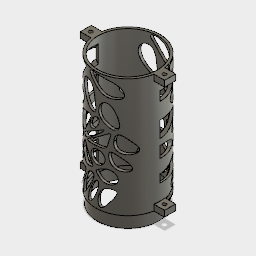
MIDDLEv2 v0XXX (Autodesk Fusion 360 design; units mm, degrees)
Autodesk Fusion 360 part; units mm, degrees
note: some values were not read from the file. Chosen so that the rebuilt part matches the saved one: that a step has no effect; which bodies a step acts on.
(part 1 of 3)
sketch "Sketch1" plane through (0, 0, 0) normal (0, 1, 0) x (1, 0, 0)
  circle A0 centre (0, 0) radius 25
  circle A1 centre (0, 0) radius 27
  circle A2 centre (0, 0) radius 26
  line L0 (-26.5898, 4.6885) -> (-35.5898, 4.6885)
  line L1 (-26.5898, -4.6885) -> (-35.5898, -4.6885)
  line L2 (-35.5898, 4.6885) -> (-35.5898, -4.6885)
  line L3 (0, 0) -> (26.3565, 0) construction
  line L4 (26.5898, 4.6885) -> (35.5898, 4.6885)
  line L5 (26.5898, -4.6885) -> (35.5898, -4.6885)
  line L6 (35.5898, -4.6885) -> (35.5898, 4.6885)
  line L7 (35.5898, 4.6885) -> (35.5898, -0.3115)
  line L8 (35.5898, -0.3115) -> (31.0898, -0.3115)
  line L9 (-35.5898, 4.6885) -> (-35.5898, -0.3115)
  line L10 (-35.5898, -0.3115) -> (-31.0898, -0.3115)
  circle A3 centre (-31.0898, -0.3115) radius 1.5
  circle A4 centre (31.0898, -0.3115) radius 1.5
extrude "Extrude1" add sketch "Sketch1" against normal blind 10 contours A2 makes body 1
extrude "Extrude2" add sketch "Sketch1" along normal blind 100 separate body contours A1 | A2 makes body 2
extrude "Extrude3" add sketch "Sketch1" along normal blind 5 separate body contours A1 L4 L5 L6 L7 | A1 L0 L1 L2 L9 makes body 3 at (31.0524, 5, -3.5204) makes body 4 at (-31.1272, 0, -3.5204)
extrude "Extrude4" cut 1 faces at (31.0524, 5, -3.5204) along direction (0, -1, 0) blind 5 on bodies 3 bodies 3
extrude "Extrude5" add sketch "Sketch1" along normal blind 100 contours A1 L4 L5 L6 L7 bodies 1 2 4
extrude "Extrude6" cut sketch "Sketch1" along normal blind 95 contours A1 L4 L5 L6 L7 bodies 2
extrude "Extrude7" add sketch "Sketch1" along normal blind 5 contours A1 L4 L5 L6 L7 bodies 2
extrude "Extrude8" cut sketch "Sketch1" along normal blind 5 contours A1 L0 L1 L2 L9 bodies 4
extrude "Extrude9" add sketch "Sketch1" along normal blind 100 contours A1 L0 L1 L2 L9 bodies 1 2
extrude "Extrude10" cut sketch "Sketch1" along normal blind 95 contours A1 L0 L1 L2 L9 bodies 2
extrude "Extrude11" add sketch "Sketch1" along normal blind 5 contours A1 L0 L1 L2 L9 bodies 2
replace_face "ReplaceFace1" [no effect]
mesh "Mesh1" [no effect]
sketch "Voronoi - Sketch2" plane through (0, 0, 0) normal (0, 0, 1) x (1, 0, 0)
  spline S0 degree 5 poles (72.3415, 4.2484) (72.4082, 4.3865) (72.5984, 4.6454) (73.0509, 4.9752) (73.962, 5.2758) (75.4951, 5.3871) (77.2684, 5.2236) (79.1091, 4.7979) (80.8407, 4.1464) (82.2997, 3.3318) (83.3471, 2.4369) (83.8777, 1.5524) (83.8316, 0.7678) (83.2057, 0.1602) (82.0668, -0.2155) (80.5337, -0.3268) (78.7604, -0.1633) (76.9197, 0.2623) (75.1881, 0.9139) (73.7291, 1.7284) (72.6817, 2.6234) (72.2572, 3.3309) (72.1984, 3.8167) (72.2749, 4.1103) (72.3415, 4.2484) knots 0 0 0 0 0 0 0.05 0.1 0.15 0.2 0.25 0.3 0.35 0.4 0.45 0.5 0.55 0.6 0.65 0.7 0.75 0.8 0.85 0.9 0.95 1 1 1 1 1 1
  spline S1 degree 5 poles (46.3148, 2.7293) (46.337, 2.8682) (46.4367, 3.1463) (46.7508, 3.5578) (47.4808, 4.0684) (48.815, 4.5828) (50.4367, 4.9223) (52.1886, 5.0509) (53.9042, 4.9524) (55.421, 4.6371) (56.5931, 4.1395) (57.3025, 3.5104) (57.4721, 2.8117) (57.0782, 2.1102) (56.1658, 1.4718) (54.8316, 0.9575) (53.2099, 0.618) (51.4579, 0.4893) (49.7424, 0.5878) (48.2256, 0.9031) (47.0535, 1.4008) (46.4859, 1.904) (46.3032, 2.3128) (46.2925, 2.5904) (46.3148, 2.7293) knots 0 0 0 0 0 0 0.05 0.1 0.15 0.2 0.25 0.3 0.35 0.4 0.45 0.5 0.55 0.6 0.65 0.7 0.75 0.8 0.85 0.9 0.95 1 1 1 1 1 1
  spline S2 degree 5 poles (90.4982, 7.9713) (90.7384, 8.2375) (91.2179, 8.7662) (91.9267, 9.5441) (92.8297, 10.5357) (93.8765, 11.6727) (94.8535, 12.6841) (95.7813, 13.5418) (96.6728, 14.207) (97.5157, 14.6194) (98.2635, 14.6976) (98.8599, 14.3734) (99.2596, 13.6216) (99.4483, 12.4904) (99.432, 11.0769) (99.2268, 9.5051) (98.8489, 7.9027) (98.3044, 6.3793) (97.579, 5.0034) (96.6518, 3.8123) (95.5082, 2.8218) (94.1538, 2.035) (92.6267, 1.4513) (91.0135, 1.0766) (89.4568, 0.9294) (88.1201, 1.0316) (87.1574, 1.4004) (86.6833, 2.0404) (86.7368, 2.9339) (87.2654, 4.0371) (88.1609, 5.2904) (89.0607, 6.3596) (89.7768, 7.1693) (90.258, 7.7052) (90.4982, 7.9713) knots 0 0 0 0 0 0 0.033333 0.066667 0.1 0.133333 0.166667 0.2 0.233333 0.266667 0.3 0.333333 0.366667 0.4 0.433333 0.466667 0.5 0.533333 0.566667 0.6 0.633333 0.666667 0.7 0.733333 0.766667 0.8 0.833333 0.866667 0.9 0.933333 0.966667 1 1 1 1 1 1
  spline S3 degree 5 poles (41.8576, 8.6332) (42.0475, 9.0262) (42.4323, 9.8124) (43.0168, 10.976) (43.7881, 12.4263) (44.7081, 13.9003) (45.5694, 14.8884) (46.3642, 15.2901) (47.083, 15.0691) (47.7037, 14.2835) (48.1907, 13.0747) (48.5028, 11.6193) (48.598, 10.0934) (48.4404, 8.6303) (48.0059, 7.285) (47.2874, 6.0631) (46.3009, 4.9442) (45.0912, 3.9084) (43.7371, 2.9591) (42.3613, 2.153) (41.1092, 1.5828) (40.1213, 1.3501) (39.5091, 1.5424) (39.3259, 2.2057) (39.55, 3.3263) (40.1114, 4.8434) (40.7519, 6.2937) (41.2925, 7.4546) (41.6676, 8.2403) (41.8576, 8.6332) knots 0 0 0 0 0 0 0.04 0.08 0.12 0.16 0.2 0.24 0.28 0.32 0.36 0.4 0.44 0.48 0.52 0.56 0.6 0.64 0.68 0.72 0.76 0.8 0.84 0.88 0.92 0.96 1 1 1 1 1 1
  spline S4 degree 5 poles (51.1992, 14.78) (51.3166, 14.7901) (51.5593, 14.7689) (51.9419, 14.6132) (52.4643, 14.1659) (53.0742, 13.268) (53.58, 12.1218) (53.93, 10.8378) (54.0877, 9.5375) (54.0399, 8.3441) (53.7944, 7.3733) (53.3764, 6.7228) (52.8255, 6.4623) (52.1932, 6.6219) (51.5401, 7.1811) (50.9302, 8.079) (50.4244, 9.2252) (50.0744, 10.5091) (49.9167, 11.8095) (49.9645, 13.0028) (50.21, 13.9737) (50.5444, 14.494) (50.855, 14.7088) (51.0818, 14.77) (51.1992, 14.78) knots 0 0 0 0 0 0 0.05 0.1 0.15 0.2 0.25 0.3 0.35 0.4 0.45 0.5 0.55 0.6 0.65 0.7 0.75 0.8 0.85 0.9 0.95 1 1 1 1 1 1
  spline S5 degree 5 poles (76.6274, 11.9383) (76.6372, 12.173) (76.695, 12.6311) (76.8959, 13.2798) (77.3869, 14.0619) (78.3402, 14.9156) (79.5819, 15.6646) (81.0431, 16.3133) (82.6365, 16.8224) (84.2611, 17.1145) (85.8113, 17.1022) (87.1843, 16.7107) (88.2878, 15.9002) (89.0488, 14.6948) (89.4192, 13.1895) (89.3745, 11.5212) (88.9153, 9.8484) (88.0682, 8.3286) (86.8872, 7.0949) (85.4537, 6.2384) (83.866, 5.8125) (82.2311, 5.8331) (80.6564, 6.2796) (79.2407, 7.0949) (78.0656, 8.1849) (77.195, 9.4353) (76.7786, 10.4711) (76.6361, 11.2226) (76.6176, 11.7035) (76.6274, 11.9383) knots 0 0 0 0 0 0 0.04 0.08 0.12 0.16 0.2 0.24 0.28 0.32 0.36 0.4 0.44 0.48 0.52 0.56 0.6 0.64 0.68 0.72 0.76 0.8 0.84 0.88 0.92 0.96 1 1 1 1 1 1
  spline S6 degree 5 poles (63.4479, 5.5707) (63.4765, 5.8196) (63.5586, 6.3186) (63.7559, 7.0631) (64.1633, 8.0259) (64.8897, 9.157) (65.799, 10.2126) (66.848, 11.1957) (67.9864, 12.1029) (69.1584, 12.9105) (70.3047, 13.5634) (71.367, 13.9945) (72.2924, 14.1422) (73.0371, 13.9685) (73.5718, 13.4785) (73.8847, 12.7343) (73.9769, 11.8229) (73.858, 10.8318) (73.5415, 9.8153) (73.0424, 8.7851) (72.3787, 7.7324) (71.5719, 6.6433) (70.6476, 5.5163) (69.6371, 4.3784) (68.5773, 3.305) (67.5102, 2.3997) (66.48, 1.772) (65.5316, 1.514) (64.7086, 1.6806) (64.0514, 2.2613) (63.5952, 3.1783) (63.4129, 4.0923) (63.3868, 4.8254) (63.4193, 5.3218) (63.4479, 5.5707) knots 0 0 0 0 0 0 0.033333 0.066667 0.1 0.133333 0.166667 0.2 0.233333 0.266667 0.3 0.333333 0.366667 0.4 0.433333 0.466667 0.5 0.533333 0.566667 0.6 0.633333 0.666667 0.7 0.733333 0.766667 0.8 0.833333 0.866667 0.9 0.933333 0.966667 1 1 1 1 1 1
  spline S7 degree 5 poles (56.2391, 14.7614) (56.3796, 14.8244) (56.6783, 14.9116) (57.1735, 14.9243) (57.8994, 14.7106) (58.8258, 14.1211) (59.6794, 13.2948) (60.3836, 12.3192) (60.8957, 11.258) (61.2184, 10.1355) (61.3834, 8.9553) (61.4387, 7.7146) (61.4339, 6.4203) (61.4083, 5.1026) (61.3747, 3.8349) (61.3136, 2.7358) (61.1898, 1.9311) (60.9656, 1.5239) (60.6136, 1.5634) (60.1323, 2.0068) (59.5414, 2.7481) (58.8736, 3.6613) (58.1676, 4.6356) (57.4602, 5.6209) (56.7855, 6.6161) (56.1757, 7.6458) (55.6622, 8.7411) (55.2755, 9.9178) (55.0461, 11.1574) (55.0053, 12.3835) (55.1783, 13.4853) (55.4975, 14.1725) (55.8349, 14.5337) (56.0985, 14.6984) (56.2391, 14.7614) knots 0 0 0 0 0 0 0.033333 0.066667 0.1 0.133333 0.166667 0.2 0.233333 0.266667 0.3 0.333333 0.366667 0.4 0.433333 0.466667 0.5 0.533333 0.566667 0.6 0.633333 0.666667 0.7 0.733333 0.766667 0.8 0.833333 0.866667 0.9 0.933333 0.966667 1 1 1 1 1 1
  spline S8 degree 5 poles (61.0368, 18.4704) (61.1208, 18.609) (61.3078, 18.8693) (61.6428, 19.2053) (62.1812, 19.5353) (62.9537, 19.7535) (63.7734, 19.7981) (64.599, 19.7002) (65.4145, 19.4945) (66.2285, 19.213) (67.0573, 18.8844) (67.9116, 18.5307) (68.7828, 18.1654) (69.626, 17.7905) (70.3559, 17.3959) (70.875, 16.9678) (71.0954, 16.494) (70.9632, 15.9714) (70.4822, 15.4119) (69.7, 14.84) (68.6922, 14.2891) (67.5473, 13.7987) (66.3526, 13.4108) (65.1778, 13.1676) (64.0739, 13.1066) (63.0787, 13.2557) (62.2201, 13.628) (61.5198, 14.2171) (60.9964, 14.9914) (60.6699, 15.8889) (60.5562, 16.8301) (60.6422, 17.5505) (60.8043, 18.0379) (60.9529, 18.3318) (61.0368, 18.4704) knots 0 0 0 0 0 0 0.033333 0.066667 0.1 0.133333 0.166667 0.2 0.233333 0.266667 0.3 0.333333 0.366667 0.4 0.433333 0.466667 0.5 0.533333 0.566667 0.6 0.633333 0.666667 0.7 0.733333 0.766667 0.8 0.833333 0.866667 0.9 0.933333 0.966667 1 1 1 1 1 1
  spline S9 degree 5 poles (32.2529, 10.7085) (32.3712, 11.1444) (32.6405, 12.0022) (33.1409, 13.2292) (33.9906, 14.692) (35.3111, 16.1518) (36.8244, 17.2073) (38.4447, 17.8567) (40.0668, 18.1217) (41.5633, 18.0377) (42.794, 17.6448) (43.634, 16.9795) (43.9948, 16.0686) (43.855, 14.9175) (43.2578, 13.5197) (42.2866, 11.8774) (41.0486, 10.0208) (39.6561, 8.0251) (38.2059, 6.0369) (36.7761, 4.2556) (35.4315, 2.8924) (34.2256, 2.1368) (33.2044, 2.12) (32.4094, 2.8766) (31.88, 4.3135) (31.6496, 6.2543) (31.724, 8.0314) (31.9305, 9.3864) (32.1345, 10.2725) (32.2529, 10.7085) knots 0 0 0 0 0 0 0.04 0.08 0.12 0.16 0.2 0.24 0.28 0.32 0.36 0.4 0.44 0.48 0.52 0.56 0.6 0.64 0.68 0.72 0.76 0.8 0.84 0.88 0.92 0.96 1 1 1 1 1 1
  spline S10 degree 5 poles (24.8243, 12.2129) (25.0629, 12.7872) (25.5668, 13.9282) (26.3917, 15.5897) (27.5776, 17.5972) (29.0561, 19.5199) (30.3822, 20.6633) (31.4217, 20.9022) (32.0705, 20.2003) (32.2714, 18.6347) (32.0115, 16.3723) (31.3173, 13.6415) (30.2519, 10.7086) (28.9128, 7.8529) (27.4305, 5.3435) (25.952, 3.4208) (24.6259, 2.2774) (23.5863, 2.0385) (22.9376, 2.7404) (22.7367, 4.306) (22.9966, 6.5684) (23.552, 8.753) (24.1355, 10.4825) (24.5858, 11.6386) (24.8243, 12.2129) knots 0 0 0 0 0 0 0.05 0.1 0.15 0.2 0.25 0.3 0.35 0.4 0.45 0.5 0.55 0.6 0.65 0.7 0.75 0.8 0.85 0.9 0.95 1 1 1 1 1 1
  spline S11 degree 5 poles (17.268, 13.2331) (17.4631, 13.7893) (17.8687, 14.8946) (18.5194, 16.5113) (19.461, 18.5209) (20.7492, 20.6827) (22.1359, 22.4285) (23.5922, 23.7207) (25.0596, 24.5397) (26.4298, 24.8708) (27.5424, 24.6968) (28.2371, 24.0071) (28.403, 22.8042) (28.0159, 21.1109) (27.1146, 18.9753) (25.7873, 16.4759) (24.1552, 13.7276) (22.3577, 10.8871) (20.537, 8.163) (18.8282, 5.7922) (17.3523, 4.0067) (16.207, 3.0022) (15.4587, 2.9065) (15.1332, 3.7451) (15.2078, 5.4125) (15.6289, 7.7162) (16.187, 9.8746) (16.6983, 11.557) (17.073, 12.6768) (17.268, 13.2331) knots 0 0 0 0 0 0 0.04 0.08 0.12 0.16 0.2 0.24 0.28 0.32 0.36 0.4 0.44 0.48 0.52 0.56 0.6 0.64 0.68 0.72 0.76 0.8 0.84 0.88 0.92 0.96 1 1 1 1 1 1
  spline S12 degree 5 poles (10.3102, 20.9494) (10.8149, 21.2169) (11.8334, 21.7299) (13.366, 22.4285) (15.3237, 23.1862) (17.383, 23.7283) (18.844, 23.7452) (19.5639, 23.1402) (19.5161, 21.8738) (18.7947, 19.9786) (17.5618, 17.5474) (16.0098, 14.7289) (14.3206, 11.7199) (12.6189, 8.7638) (10.9563, 6.1332) (9.3453, 4.0908) (7.7798, 2.8557) (6.2615, 2.5656) (4.8231, 3.2424) (3.5554, 4.7485) (2.5835, 6.8422) (2.0391, 9.242) (2.0349, 11.6812) (2.6343, 13.9797) (3.8378, 16.0625) (5.5922, 17.9151) (7.3525, 19.2278) (8.8048, 20.1248) (9.8054, 20.6819) (10.3102, 20.9494) knots 0 0 0 0 0 0 0.04 0.08 0.12 0.16 0.2 0.24 0.28 0.32 0.36 0.4 0.44 0.48 0.52 0.56 0.6 0.64 0.68 0.72 0.76 0.8 0.84 0.88 0.92 0.96 1 1 1 1 1 1
  spline S13 degree 5 poles (47.6318, 23.3164) (47.71, 23.5584) (47.8666, 24.0455) (48.0999, 24.7784) (48.4055, 25.7323) (48.7925, 26.8161) (49.2107, 27.7272) (49.6905, 28.4126) (50.2587, 28.8365) (50.93, 28.9852) (51.6992, 28.8738) (52.5452, 28.5385) (53.4369, 28.0279) (54.3384, 27.3945) (55.2143, 26.6868) (56.0354, 25.9399) (56.7807, 25.1733) (57.4342, 24.3969) (57.9833, 23.6149) (58.4166, 22.8301) (58.7222, 22.048) (58.885, 21.2818) (58.8885, 20.5523) (58.7198, 19.8808) (58.3746, 19.2849) (57.8623, 18.7723) (57.2098, 18.3367) (56.4548, 17.9646) (55.6393, 17.6413) (54.8035, 17.3571) (53.979, 17.1138) (53.1838, 16.9293) (52.4252, 16.8266) (51.7018, 16.8247) (51.0065, 16.9298) (50.3281, 17.1237) (49.6548, 17.3629) (48.9811, 17.5999) (48.3137, 17.7997) (47.6774, 17.9571) (47.1223, 18.1157) (46.7059, 18.3456) (46.4753, 18.719) (46.4452, 19.2835) (46.5929, 20.0505) (46.8749, 21.0047) (47.1654, 21.8879) (47.3973, 22.5935) (47.5536, 23.0744) (47.6318, 23.3164) knots 0 0 0 0 0 0 0.022222 0.044444 0.066667 0.088889 0.111111 0.133333 0.155556 0.177778 0.2 0.222222 0.244444 0.266667 0.288889 0.311111 0.333333 0.355556 0.377778 0.4 0.422222 0.444444 0.466667 0.488889 0.511111 0.533333 0.555556 0.577778 0.6 0.622222 0.644444 0.666667 0.688889 0.711111 0.733333 0.755556 0.777778 0.8 0.822222 0.844444 0.866667 0.888889 0.911111 0.933333 0.955556 0.977778 1 1 1 1 1 1
  spline S14 degree 5 poles (74.4124, 23.0453) (74.4913, 23.297) (74.6533, 23.8002) (74.9079, 24.548) (75.2692, 25.5032) (75.7612, 26.5584) (76.3004, 27.4119) (76.8928, 28.0144) (77.5397, 28.3362) (78.2344, 28.3754) (78.9584, 28.1616) (79.6858, 27.7425) (80.3851, 27.1717) (81.0227, 26.4977) (81.5653, 25.7499) (81.9819, 24.9416) (82.2458, 24.0785) (82.3363, 23.1652) (82.2407, 22.2113) (81.9561, 21.2404) (81.4897, 20.2874) (80.8579, 19.3915) (80.0855, 18.5911) (79.2048, 17.9177) (78.2555, 17.3903) (77.2839, 17.0086) (76.3389, 16.7611) (75.4678, 16.6321) (74.7122, 16.6099) (74.104, 16.6934) (73.6606, 16.9024) (73.3853, 17.268) (73.271, 17.8184) (73.3013, 18.5636) (73.4538, 19.493) (73.7038, 20.5795) (73.9622, 21.541) (74.1797, 22.2901) (74.3335, 22.7936) (74.4124, 23.0453) knots 0 0 0 0 0 0 0.028571 0.057143 0.085714 0.114286 0.142857 0.171429 0.2 0.228571 0.257143 0.285714 0.314286 0.342857 0.371429 0.4 0.428571 0.457143 0.485714 0.514286 0.542857 0.571429 0.6 0.628571 0.657143 0.685714 0.714286 0.742857 0.771429 0.8 0.828571 0.857143 0.885714 0.914286 0.942857 0.971429 1 1 1 1 1 1
  spline S15 degree 5 poles (68.4437, 26.228) (68.531, 26.5376) (68.7289, 27.1443) (69.0917, 28.0013) (69.6843, 28.9818) (70.5311, 29.8189) (71.3981, 30.1819) (72.1992, 30.0272) (72.8573, 29.3655) (73.3127, 28.2684) (73.5233, 26.8493) (73.4675, 25.2495) (73.1466, 23.6242) (72.5875, 22.1282) (71.8467, 20.9026) (70.9999, 20.0655) (70.1329, 19.7024) (69.3319, 19.8572) (68.6737, 20.5189) (68.2184, 21.6159) (68.0078, 23.0351) (68.0523, 24.3149) (68.2051, 25.2863) (68.3564, 25.9183) (68.4437, 26.228) knots 0 0 0 0 0 0 0.05 0.1 0.15 0.2 0.25 0.3 0.35 0.4 0.45 0.5 0.55 0.6 0.65 0.7 0.75 0.8 0.85 0.9 0.95 1 1 1 1 1 1
  spline S16 degree 5 poles (6.8565, 26.1554) (7.2699, 26.3826) (8.1115, 26.8214) (9.3992, 27.4216) (11.0839, 28.0667) (12.9317, 28.54) (14.3369, 28.6331) (15.1534, 28.3316) (15.293, 27.6579) (14.7486, 26.6793) (13.5843, 25.4968) (11.9185, 24.2299) (9.9114, 23.0046) (7.752, 21.9396) (5.6461, 21.1331) (3.7982, 20.6599) (2.3931, 20.5668) (1.5766, 20.8683) (1.437, 21.542) (1.9814, 22.5205) (3.1457, 23.7031) (4.4783, 24.7166) (5.6314, 25.458) (6.4431, 25.9281) (6.8565, 26.1554) knots 0 0 0 0 0 0 0.05 0.1 0.15 0.2 0.25 0.3 0.35 0.4 0.45 0.5 0.55 0.6 0.65 0.7 0.75 0.8 0.85 0.9 0.95 1 1 1 1 1 1
  spline S17 degree 5 poles (86.9545, 28.4347) (87.1266, 28.6316) (87.4812, 29.0114) (88.0387, 29.5327) (88.8141, 30.0994) (89.7947, 30.5153) (90.7534, 30.5731) (91.6677, 30.2315) (92.5291, 29.489) (93.3384, 28.382) (94.0981, 26.9755) (94.8057, 25.3569) (95.4464, 23.6287) (95.9857, 21.9017) (96.3639, 20.2883) (96.5121, 18.8927) (96.3668, 17.8016) (95.8843, 17.0748) (95.0558, 16.7354) (93.9232, 16.7593) (92.5655, 17.0897) (91.0849, 17.6522) (89.5915, 18.3707) (88.1908, 19.1811) (86.9675, 20.0487) (85.9847, 20.9622) (85.2849, 21.9239) (84.8902, 22.9405) (84.8023, 24.0154) (85.0025, 25.1381) (85.4554, 26.283) (85.983, 27.1852) (86.4483, 27.8305) (86.7823, 28.2379) (86.9545, 28.4347) knots 0 0 0 0 0 0 0.033333 0.066667 0.1 0.133333 0.166667 0.2 0.233333 0.266667 0.3 0.333333 0.366667 0.4 0.433333 0.466667 0.5 0.533333 0.566667 0.6 0.633333 0.666667 0.7 0.733333 0.766667 0.8 0.833333 0.866667 0.9 0.933333 0.966667 1 1 1 1 1 1
  spline S18 degree 5 poles (30.268, 27.4809) (30.2888, 27.5763) (30.3595, 27.7733) (30.558, 28.0901) (31.0122, 28.5606) (31.8627, 29.2146) (32.9338, 29.8998) (34.1511, 30.5669) (35.446, 31.158) (36.7693, 31.6125) (38.0846, 31.8728) (39.364, 31.8903) (40.5828, 31.6308) (41.7145, 31.0806) (42.7259, 30.2527) (43.5724, 29.1919) (44.206, 27.9652) (44.5813, 26.653) (44.6625, 25.3403) (44.4303, 24.1087) (43.8886, 23.0264) (43.0708, 22.1413) (42.03, 21.4838) (40.8324, 21.0681) (39.5495, 20.8943) (38.2507, 20.9501) (36.9952, 21.2122) (35.8286, 21.6486) (34.7824, 22.2211) (33.8737, 22.887) (33.1035, 23.6019) (32.4562, 24.3216) (31.8982, 25.0047) (31.3954, 25.619) (30.9313, 26.1493) (30.523, 26.6037) (30.3, 26.9395) (30.235, 27.2009) (30.2472, 27.3855) (30.268, 27.4809) knots 0 0 0 0 0 0 0.028571 0.057143 0.085714 0.114286 0.142857 0.171429 0.2 0.228571 0.257143 0.285714 0.314286 0.342857 0.371429 0.4 0.428571 0.457143 0.485714 0.514286 0.542857 0.571429 0.6 0.628571 0.657143 0.685714 0.714286 0.742857 0.771429 0.8 0.828571 0.857143 0.885714 0.914286 0.942857 0.971429 1 1 1 1 1 1
  spline S19 degree 5 poles (63.3984, 29.454) (63.5581, 29.6534) (63.8804, 30.0484) (64.3678, 30.625) (65.0078, 31.343) (65.7591, 32.1004) (66.4382, 32.663) (67.028, 32.9865) (67.5153, 33.0443) (67.8871, 32.84) (68.1323, 32.4027) (68.2461, 31.7706) (68.2354, 30.9756) (68.1167, 30.0419) (67.9101, 28.9926) (67.6352, 27.8544) (67.306, 26.6625) (66.9254, 25.4661) (66.4817, 24.3324) (65.9582, 23.3354) (65.3405, 22.547) (64.6263, 22.0261) (63.8318, 21.8104) (63.0038, 21.903) (62.2184, 22.2721) (61.5608, 22.8656) (61.1096, 23.6233) (60.9207, 24.4891) (61.0075, 25.4252) (61.3492, 26.4074) (61.9006, 27.4189) (62.4622, 28.2392) (62.9225, 28.8516) (63.2387, 29.2545) (63.3984, 29.454) knots 0 0 0 0 0 0 0.033333 0.066667 0.1 0.133333 0.166667 0.2 0.233333 0.266667 0.3 0.333333 0.366667 0.4 0.433333 0.466667 0.5 0.533333 0.566667 0.6 0.633333 0.666667 0.7 0.733333 0.766667 0.8 0.833333 0.866667 0.9 0.933333 0.966667 1 1 1 1 1 1
  spline S20 degree 5 poles (53.3845, 32.2911) (53.4094, 32.411) (53.4975, 32.64) (53.745, 32.9504) (54.2992, 33.3048) (55.3125, 33.6931) (56.5672, 34.0763) (57.9672, 34.4881) (59.4086, 34.9224) (60.788, 35.3156) (62.009, 35.5753) (62.9884, 35.604) (63.6631, 35.3253) (63.9961, 34.7073) (63.9853, 33.7937) (63.6567, 32.6863) (63.0548, 31.5172) (62.234, 30.4259) (61.2501, 29.5341) (60.151, 28.9199) (58.9801, 28.6197) (57.7803, 28.6348) (56.5991, 28.9365) (55.4921, 29.4706) (54.5295, 30.1613) (53.7928, 30.92) (53.4456, 31.5133) (53.3483, 31.9207) (53.3597, 32.1712) (53.3845, 32.2911) knots 0 0 0 0 0 0 0.04 0.08 0.12 0.16 0.2 0.24 0.28 0.32 0.36 0.4 0.44 0.48 0.52 0.56 0.6 0.64 0.68 0.72 0.76 0.8 0.84 0.88 0.92 0.96 1 1 1 1 1 1
  spline S21 degree 5 poles (95.2862, 31.8833) (95.3888, 32.0426) (95.6243, 32.3364) (96.0604, 32.6994) (96.7572, 33.0092) (97.6575, 33.0488) (98.4324, 32.6906) (98.9947, 31.9106) (99.3374, 30.7196) (99.5011, 29.1603) (99.5542, 27.3078) (99.568, 25.2698) (99.5942, 23.1868) (99.6422, 21.2327) (99.6917, 19.5899) (99.7039, 18.4253) (99.6333, 17.865) (99.4384, 17.9724) (99.0944, 18.7146) (98.5972, 19.9783) (97.9628, 21.6035) (97.2296, 23.4132) (96.4577, 25.2411) (95.7337, 26.9665) (95.1619, 28.5237) (94.8413, 29.8803) (94.8457, 30.7949) (95.0088, 31.3807) (95.1836, 31.724) (95.2862, 31.8833) knots 0 0 0 0 0 0 0.04 0.08 0.12 0.16 0.2 0.24 0.28 0.32 0.36 0.4 0.44 0.48 0.52 0.56 0.6 0.64 0.68 0.72 0.76 0.8 0.84 0.88 0.92 0.96 1 1 1 1 1 1
  spline S22 degree 5 poles (14.9018, 34.94) (14.8985, 35.1162) (14.9102, 35.47) (14.9811, 36.0055) (15.1698, 36.7332) (15.5134, 37.6701) (15.9084, 38.6315) (16.303, 39.6017) (16.6602, 40.55) (16.9719, 41.4234) (17.2587, 42.1525) (17.5529, 42.6694) (17.8872, 42.9213) (18.2783, 42.8893) (18.7204, 42.5951) (19.2011, 42.0795) (19.7144, 41.3837) (20.2699, 40.5361) (20.8833, 39.5588) (21.5709, 38.4704) (22.3427, 37.2899) (23.1952, 36.0411) (24.1059, 34.7556) (25.0242, 33.478) (25.8755, 32.2633) (26.5772, 31.167) (27.0506, 30.2372) (27.2352, 29.5062) (27.1005, 28.9826) (26.6623, 28.6413) (25.9892, 28.42) (25.1754, 28.2456) (24.3174, 28.056) (23.489, 27.8249) (22.7185, 27.5823) (22.0033, 27.3907) (21.3221, 27.3221) (20.6468, 27.4376) (19.9566, 27.7604) (19.2421, 28.2769) (18.5044, 28.9507) (17.7557, 29.734) (17.0189, 30.5782) (16.3291, 31.4475) (15.7294, 32.3221) (15.2625, 33.1937) (15.0238, 33.8892) (14.9299, 34.4127) (14.905, 34.7638) (14.9018, 34.94) knots 0 0 0 0 0 0 0.022222 0.044444 0.066667 0.088889 0.111111 0.133333 0.155556 0.177778 0.2 0.222222 0.244444 0.266667 0.288889 0.311111 0.333333 0.355556 0.377778 0.4 0.422222 0.444444 0.466667 0.488889 0.511111 0.533333 0.555556 0.577778 0.6 0.622222 0.644444 0.666667 0.688889 0.711111 0.733333 0.755556 0.777778 0.8 0.822222 0.844444 0.866667 0.888889 0.911111 0.933333 0.955556 0.977778 1 1 1 1 1 1
  spline S23 degree 5 poles (7.035, 34.851) (7.3775, 35.0049) (8.0604, 35.2761) (9.0625, 35.565) (10.2878, 35.694) (11.4821, 35.4162) (12.2154, 34.7258) (12.4072, 33.6852) (12.0411, 32.3938) (11.1629, 30.979) (9.8643, 29.5805) (8.272, 28.3373) (6.5362, 27.3738) (4.8199, 26.7854) (3.2883, 26.6241) (2.094, 26.9019) (1.3607, 27.5923) (1.1689, 28.6329) (1.535, 29.9243) (2.4132, 31.3392) (3.7119, 32.7377) (4.9857, 33.7322) (6.0056, 34.3523) (6.6925, 34.697) (7.035, 34.851) knots 0 0 0 0 0 0 0.05 0.1 0.15 0.2 0.25 0.3 0.35 0.4 0.45 0.5 0.55 0.6 0.65 0.7 0.75 0.8 0.85 0.9 0.95 1 1 1 1 1 1
  spline S24 degree 5 poles (80.8897, 35.467) (80.9358, 35.7693) (81.038, 36.3722) (81.2189, 37.2603) (81.5122, 38.3646) (81.9688, 39.4949) (82.5218, 40.2734) (83.1714, 40.6281) (83.9033, 40.5294) (84.6783, 40.0076) (85.4398, 39.1366) (86.1228, 38.0158) (86.6624, 36.752) (87.0023, 35.4423) (87.1039, 34.1564) (86.9473, 32.9445) (86.5332, 31.844) (85.8847, 30.8866) (85.0492, 30.1047) (84.1026, 29.5399) (83.1398, 29.2398) (82.2561, 29.2461) (81.533, 29.5872) (81.0192, 30.2667) (80.7214, 31.2576) (80.6203, 32.5077) (80.6688, 33.6558) (80.7611, 34.5586) (80.8435, 35.1648) (80.8897, 35.467) knots 0 0 0 0 0 0 0.04 0.08 0.12 0.16 0.2 0.24 0.28 0.32 0.36 0.4 0.44 0.48 0.52 0.56 0.6 0.64 0.68 0.72 0.76 0.8 0.84 0.88 0.92 0.96 1 1 1 1 1 1
  spline S25 degree 5 poles (73.0612, 37.9814) (73.2662, 38.1894) (73.6812, 38.6033) (74.3118, 39.2105) (75.1437, 39.9578) (76.1194, 40.6959) (76.9939, 41.1532) (77.7412, 41.2631) (78.345, 40.9885) (78.7981, 40.3357) (79.1006, 39.3539) (79.2577, 38.1222) (79.2779, 36.7396) (79.1706, 35.3148) (78.9447, 33.9554) (78.6063, 32.7586) (78.1604, 31.8042) (77.6109, 31.1471) (76.9616, 30.8106) (76.217, 30.7778) (75.3828, 30.9848) (74.4714, 31.3431) (73.5071, 31.7612) (72.5305, 32.1656) (71.6059, 32.5261) (70.8205, 32.8661) (70.2625, 33.2363) (70.0045, 33.6967) (70.0829, 34.2932) (70.4841, 35.0415) (71.1606, 35.9319) (71.8659, 36.7313) (72.4513, 37.3557) (72.8562, 37.7735) (73.0612, 37.9814) knots 0 0 0 0 0 0 0.033333 0.066667 0.1 0.133333 0.166667 0.2 0.233333 0.266667 0.3 0.333333 0.366667 0.4 0.433333 0.466667 0.5 0.533333 0.566667 0.6 0.633333 0.666667 0.7 0.733333 0.766667 0.8 0.833333 0.866667 0.9 0.933333 0.966667 1 1 1 1 1 1
  spline S26 degree 5 poles (1.5577, 56.6899) (1.6941, 56.7347) (1.9941, 56.7534) (2.5249, 56.5723) (3.3897, 55.9536) (4.7011, 54.7284) (6.1945, 53.2614) (7.8053, 51.7558) (9.4534, 50.3656) (11.0447, 49.1559) (12.4799, 48.1244) (13.663, 47.2221) (14.5111, 46.3741) (14.9625, 45.4992) (14.9872, 44.5316) (14.588, 43.4346) (13.7976, 42.2129) (12.6795, 40.9285) (11.3232, 39.7028) (9.8309, 38.6865) (8.3052, 38.035) (6.8371, 37.8833) (5.4926, 38.3177) (4.3044, 39.3576) (3.2841, 40.9659) (2.4293, 43.0552) (1.7332, 45.4938) (1.1925, 48.1131) (0.8179, 50.7106) (0.6327, 53.069) (0.6654, 54.9831) (0.8883, 56.025) (1.1755, 56.4841) (1.4212, 56.645) (1.5577, 56.6899) knots 0 0 0 0 0 0 0.033333 0.066667 0.1 0.133333 0.166667 0.2 0.233333 0.266667 0.3 0.333333 0.366667 0.4 0.433333 0.466667 0.5 0.533333 0.566667 0.6 0.633333 0.666667 0.7 0.733333 0.766667 0.8 0.833333 0.866667 0.9 0.933333 0.966667 1 1 1 1 1 1
  spline S27 degree 5 poles (89.2099, 43.4393) (89.3472, 43.543) (89.6375, 43.7233) (90.1159, 43.9101) (90.8162, 43.9878) (91.7213, 43.8095) (92.5798, 43.3816) (93.3263, 42.7418) (93.9219, 41.9346) (94.3615, 41.0084) (94.6605, 40.012) (94.8447, 38.9918) (94.9395, 37.989) (94.9599, 37.0366) (94.8982, 36.1556) (94.7319, 35.3595) (94.4364, 34.6589) (93.9949, 34.0666) (93.4114, 33.603) (92.7176, 33.299) (91.9596, 33.1873) (91.1889, 33.2966) (90.4505, 33.6441) (89.7745, 34.2289) (89.1803, 35.0347) (88.6812, 36.0303) (88.289, 37.1718) (88.0171, 38.4036) (87.8865, 39.6591) (87.9216, 40.8657) (88.1427, 41.9512) (88.477, 42.6701) (88.8137, 43.101) (89.0726, 43.3356) (89.2099, 43.4393) knots 0 0 0 0 0 0 0.033333 0.066667 0.1 0.133333 0.166667 0.2 0.233333 0.266667 0.3 0.333333 0.366667 0.4 0.433333 0.466667 0.5 0.533333 0.566667 0.6 0.633333 0.666667 0.7 0.733333 0.766667 0.8 0.833333 0.866667 0.9 0.933333 0.966667 1 1 1 1 1 1
  spline S28 degree 5 poles (29.4392, 43.2903) (29.7767, 43.4057) (30.4694, 43.5839) (31.5456, 43.6879) (32.9858, 43.4909) (34.618, 42.7175) (35.9177, 41.4947) (36.7505, 39.9379) (37.0303, 38.1919) (36.738, 36.4248) (35.9106, 34.8103) (34.6313, 33.511) (33.0209, 32.6609) (31.2294, 32.3477) (29.4292, 32.594) (27.797, 33.3674) (26.4973, 34.5902) (25.6645, 36.147) (25.3847, 37.893) (25.677, 39.6601) (26.5044, 41.2746) (27.5278, 42.3141) (28.4444, 42.8915) (29.1017, 43.1749) (29.4392, 43.2903) knots 0 0 0 0 0 0 0.05 0.1 0.15 0.2 0.25 0.3 0.35 0.4 0.45 0.5 0.55 0.6 0.65 0.7 0.75 0.8 0.85 0.9 0.95 1 1 1 1 1 1
  spline S29 degree 5 poles (40.0127, 44.8616) (40.1336, 44.932) (40.3968, 45.0372) (40.854, 45.0869) (41.5775, 44.9433) (42.6257, 44.464) (43.7606, 43.7557) (44.9222, 42.8952) (46.0547, 41.9518) (47.116, 40.971) (48.0757, 39.9785) (48.913, 38.9873) (49.6145, 38.0029) (50.1721, 37.0298) (50.5807, 36.077) (50.8363, 35.1651) (50.9345, 34.3232) (50.8702, 33.5817) (50.6368, 32.967) (50.2244, 32.494) (49.6242, 32.1665) (48.8377, 31.9833) (47.8847, 31.9426) (46.8093, 32.0463) (45.6692, 32.2982) (44.527, 32.703) (43.441, 33.2651) (42.4567, 33.9877) (41.5972, 34.8711) (40.8692, 35.9102) (40.2695, 37.0904) (39.7916, 38.3849) (39.4316, 39.7508) (39.1948, 41.1258) (39.102, 42.4242) (39.1818, 43.5511) (39.4054, 44.2438) (39.6711, 44.6146) (39.8917, 44.7912) (40.0127, 44.8616) knots 0 0 0 0 0 0 0.028571 0.057143 0.085714 0.114286 0.142857 0.171429 0.2 0.228571 0.257143 0.285714 0.314286 0.342857 0.371429 0.4 0.428571 0.457143 0.485714 0.514286 0.542857 0.571429 0.6 0.628571 0.657143 0.685714 0.714286 0.742857 0.771429 0.8 0.828571 0.857143 0.885714 0.914286 0.942857 0.971429 1 1 1 1 1 1
  spline S30 degree 5 poles (97.6808, 40.0308) (97.7875, 40.0282) (98.0026, 39.9977) (98.3253, 39.8769) (98.7348, 39.5723) (99.163, 38.9931) (99.4645, 38.2737) (99.6077, 37.4838) (99.5761, 36.6983) (99.3745, 35.9915) (99.0251, 35.4317) (98.5636, 35.0752) (98.0346, 34.9606) (97.4882, 35.1021) (96.9762, 35.4829) (96.5481, 36.0621) (96.2466, 36.7815) (96.1034, 37.5714) (96.1349, 38.3569) (96.3366, 39.0637) (96.6859, 39.6235) (97.0552, 39.9087) (97.3625, 40.0137) (97.5741, 40.0335) (97.6808, 40.0308) knots 0 0 0 0 0 0 0.05 0.1 0.15 0.2 0.25 0.3 0.35 0.4 0.45 0.5 0.55 0.6 0.65 0.7 0.75 0.8 0.85 0.9 0.95 1 1 1 1 1 1
  spline S31 degree 5 poles (54.9206, 43.9297) (55.1007, 44.1144) (55.4665, 44.4698) (56.026, 44.9586) (56.7721, 45.5153) (57.6634, 46.0511) (58.4835, 46.4324) (59.2126, 46.6646) (59.8404, 46.7471) (60.365, 46.6645) (60.7897, 46.3942) (61.1191, 45.9184) (61.3539, 45.2363) (61.4904, 44.3662) (61.5209, 43.3411) (61.4338, 42.206) (61.2137, 41.0148) (60.8419, 39.8284) (60.3017, 38.7095) (59.5843, 37.7199) (58.6943, 36.9156) (57.6555, 36.3435) (56.5171, 36.0365) (55.3594, 36.0103) (54.2787, 36.2642) (53.3728, 36.7823) (52.7265, 37.5346) (52.3971, 38.4779) (52.398, 39.5567) (52.7056, 40.7074) (53.2708, 41.865) (53.8768, 42.7475) (54.3858, 43.3617) (54.7405, 43.745) (54.9206, 43.9297) knots 0 0 0 0 0 0 0.033333 0.066667 0.1 0.133333 0.166667 0.2 0.233333 0.266667 0.3 0.333333 0.366667 0.4 0.433333 0.466667 0.5 0.533333 0.566667 0.6 0.633333 0.666667 0.7 0.733333 0.766667 0.8 0.833333 0.866667 0.9 0.933333 0.966667 1 1 1 1 1 1
  spline S32 degree 5 poles (68.339, 45.7064) (68.6278, 45.7573) (69.2123, 45.8388) (70.0998, 45.8994) (71.2593, 45.8557) (72.5519, 45.6005) (73.5797, 45.1586) (74.2584, 44.5488) (74.5392, 43.7932) (74.4275, 42.9149) (73.979, 41.9385) (73.2793, 40.8921) (72.4275, 39.8097) (71.5197, 38.733) (70.6303, 37.7141) (69.8007, 36.8152) (69.0477, 36.0988) (68.368, 35.6198) (67.744, 35.4169) (67.149, 35.5029) (66.5532, 35.8598) (65.936, 36.4503) (65.2956, 37.2262) (64.6629, 38.1395) (64.0985, 39.1455) (63.6764, 40.2016) (63.4716, 41.2672) (63.5474, 42.3027) (63.9397, 43.2694) (64.6514, 44.1298) (65.6569, 44.8496) (66.6553, 45.2896) (67.4797, 45.5332) (68.0502, 45.6554) (68.339, 45.7064) knots 0 0 0 0 0 0 0.033333 0.066667 0.1 0.133333 0.166667 0.2 0.233333 0.266667 0.3 0.333333 0.366667 0.4 0.433333 0.466667 0.5 0.533333 0.566667 0.6 0.633333 0.666667 0.7 0.733333 0.766667 0.8 0.833333 0.866667 0.9 0.933333 0.966667 1 1 1 1 1 1
  spline S33 degree 5 poles (92.6578, 47.5854) (92.7048, 47.6997) (92.825, 47.9236) (93.0837, 48.2436) (93.5749, 48.6287) (94.3778, 48.9991) (95.2956, 49.2108) (96.2466, 49.2187) (97.1521, 48.9917) (97.9464, 48.5204) (98.5767, 47.8161) (99.0054, 46.9118) (99.2118, 45.8619) (99.1941, 44.7434) (98.9721, 43.6568) (98.5802, 42.711) (98.0605, 42.0077) (97.4564, 41.6242) (96.8059, 41.5992) (96.1335, 41.9117) (95.4538, 42.4926) (94.7789, 43.2478) (94.125, 44.0783) (93.5184, 44.8991) (93.0045, 45.6634) (92.6425, 46.3616) (92.5205, 46.8738) (92.543, 47.2375) (92.6108, 47.471) (92.6578, 47.5854) knots 0 0 0 0 0 0 0.04 0.08 0.12 0.16 0.2 0.24 0.28 0.32 0.36 0.4 0.44 0.48 0.52 0.56 0.6 0.64 0.68 0.72 0.76 0.8 0.84 0.88 0.92 0.96 1 1 1 1 1 1
  spline S34 degree 5 poles (42.1469, 53.3617) (42.1704, 53.7144) (42.2377, 54.4135) (42.3961, 55.4299) (42.7146, 56.6666) (43.2889, 57.8764) (44.0438, 58.6306) (44.9808, 58.8474) (46.0873, 58.5096) (47.3319, 57.6623) (48.6648, 56.3931) (50.0163, 54.8175) (51.2968, 53.0631) (52.3931, 51.2536) (53.1783, 49.4995) (53.5364, 47.8993) (53.3826, 46.536) (52.6844, 45.4761) (51.4872, 44.7667) (49.9257, 44.4342) (48.1824, 44.4872) (46.4543, 44.9187) (44.9189, 45.7072) (43.696, 46.8192) (42.8267, 48.2093) (42.3011, 49.8186) (42.1211, 51.2214) (42.0968, 52.2968) (42.1235, 53.0089) (42.1469, 53.3617) knots 0 0 0 0 0 0 0.04 0.08 0.12 0.16 0.2 0.24 0.28 0.32 0.36 0.4 0.44 0.48 0.52 0.56 0.6 0.64 0.68 0.72 0.76 0.8 0.84 0.88 0.92 0.96 1 1 1 1 1 1
  spline S35 degree 5 poles (76.8761, 50.2318) (76.9135, 50.4324) (76.9956, 50.8353) (77.1395, 51.4436) (77.3703, 52.2597) (77.7215, 53.2871) (78.1364, 54.3188) (78.6162, 55.3437) (79.1602, 56.3363) (79.7623, 57.2488) (80.4103, 58.0095) (81.0902, 58.5411) (81.7901, 58.7761) (82.503, 58.6708) (83.2319, 58.2247) (83.9875, 57.4784) (84.7809, 56.4986) (85.6182, 55.3676) (86.4942, 54.1706) (87.3871, 52.9848) (88.2501, 51.8655) (89.0168, 50.8439) (89.6152, 49.9324) (89.9795, 49.1285) (90.0633, 48.4182) (89.8507, 47.7801) (89.3717, 47.1892) (88.6874, 46.6217) (87.8725, 46.06) (86.9998, 45.4973) (86.1213, 44.9439) (85.2597, 44.4274) (84.4199, 43.9829) (83.595, 43.6455) (82.7743, 43.4422) (81.9514, 43.3828) (81.1292, 43.4563) (80.318, 43.6419) (79.5343, 43.9172) (78.7999, 44.2667) (78.1407, 44.692) (77.5826, 45.2047) (77.1472, 45.8181) (76.8475, 46.54) (76.6829, 47.3632) (76.6415, 48.2685) (76.6932, 49.0389) (76.7713, 49.6317) (76.8387, 50.0312) (76.8761, 50.2318) knots 0 0 0 0 0 0 0.022222 0.044444 0.066667 0.088889 0.111111 0.133333 0.155556 0.177778 0.2 0.222222 0.244444 0.266667 0.288889 0.311111 0.333333 0.355556 0.377778 0.4 0.422222 0.444444 0.466667 0.488889 0.511111 0.533333 0.555556 0.577778 0.6 0.622222 0.644444 0.666667 0.688889 0.711111 0.733333 0.755556 0.777778 0.8 0.822222 0.844444 0.866667 0.888889 0.911111 0.933333 0.955556 0.977778 1 1 1 1 1 1
  spline S36 degree 5 poles (30.4058, 52.0766) (30.9134, 52.4287) (31.929, 53.1367) (33.4347, 54.1966) (35.3335, 55.5461) (37.369, 56.9664) (38.9474, 57.9697) (39.9981, 58.4371) (40.5104, 58.3014) (40.5459, 57.5698) (40.2485, 56.3439) (39.793, 54.7832) (39.3372, 53.0717) (38.971, 51.3841) (38.67, 49.8524) (38.3366, 48.5664) (37.8403, 47.5723) (37.0554, 46.8732) (35.9059, 46.4247) (34.3733, 46.1508) (32.4915, 45.9654) (30.3459, 45.7938) (28.0706, 45.5915) (25.8499, 45.3692) (23.8938, 45.1819) (22.4085, 45.1083) (21.5665, 45.2337) (21.4793, 45.6321) (22.1623, 46.3463) (23.5463, 47.3856) (25.5008, 48.7271) (27.382, 49.9983) (28.8836, 51.0241) (29.8983, 51.7245) (30.4058, 52.0766) knots 0 0 0 0 0 0 0.033333 0.066667 0.1 0.133333 0.166667 0.2 0.233333 0.266667 0.3 0.333333 0.366667 0.4 0.433333 0.466667 0.5 0.533333 0.566667 0.6 0.633333 0.666667 0.7 0.733333 0.766667 0.8 0.833333 0.866667 0.9 0.933333 0.966667 1 1 1 1 1 1
  spline S37 degree 5 poles (64.1181, 50.5536) (64.267, 50.7261) (64.5797, 51.0703) (65.0894, 51.577) (65.8399, 52.2019) (66.8857, 52.8231) (68.031, 53.2194) (69.2572, 53.346) (70.5239, 53.186) (71.7519, 52.7633) (72.8266, 52.1396) (73.6253, 51.3961) (74.0377, 50.6181) (73.9879, 49.8803) (73.462, 49.228) (72.5092, 48.6758) (71.2209, 48.2207) (69.7175, 47.8504) (68.1313, 47.5538) (66.5923, 47.3305) (65.2128, 47.2006) (64.084, 47.1947) (63.2717, 47.3448) (62.8126, 47.675) (62.7098, 48.1921) (62.9271, 48.8758) (63.3102, 49.5218) (63.6862, 50.0353) (63.9692, 50.3811) (64.1181, 50.5536) knots 0 0 0 0 0 0 0.04 0.08 0.12 0.16 0.2 0.24 0.28 0.32 0.36 0.4 0.44 0.48 0.52 0.56 0.6 0.64 0.68 0.72 0.76 0.8 0.84 0.88 0.92 0.96 1 1 1 1 1 1
  spline S38 degree 5 poles (17.7007, 48.1543) (17.7411, 48.2619) (17.8546, 48.4866) (18.1345, 48.8587) (18.7596, 49.4452) (19.977, 50.3508) (21.5946, 51.4269) (23.5354, 52.6486) (25.6928, 53.9712) (27.9417, 55.3314) (30.1495, 56.6498) (32.1837, 57.8377) (33.9197, 58.8058) (35.2483, 59.4722) (36.0837, 59.7706) (36.3706, 59.6582) (36.0944, 59.1259) (35.2836, 58.2012) (34, 56.9402) (32.3323, 55.422) (30.3884, 53.7424) (28.2886, 52.0084) (26.1587, 50.3317) (24.1227, 48.8234) (22.2922, 47.5827) (20.7564, 46.6863) (19.572, 46.1788) (18.7509, 46.0599) (18.2535, 46.2771) (17.9658, 46.7044) (17.7537, 47.1865) (17.6257, 47.5549) (17.612, 47.8411) (17.6603, 48.0467) (17.7007, 48.1543) knots 0 0 0 0 0 0 0.033333 0.066667 0.1 0.133333 0.166667 0.2 0.233333 0.266667 0.3 0.333333 0.366667 0.4 0.433333 0.466667 0.5 0.533333 0.566667 0.6 0.633333 0.666667 0.7 0.733333 0.766667 0.8 0.833333 0.866667 0.9 0.933333 0.966667 1 1 1 1 1 1
  spline S39 degree 5 poles (47.9123, 60.7108) (47.936, 60.8427) (48.03, 61.0949) (48.3098, 61.4415) (48.9398, 61.8567) (50.0542, 62.3385) (51.3726, 62.813) (52.7769, 63.2871) (54.1858, 63.7295) (55.5531, 64.0794) (56.8553, 64.2641) (58.0821, 64.2145) (59.2261, 63.8796) (60.2716, 63.2453) (61.1904, 62.3394) (61.9506, 61.2146) (62.5222, 59.9375) (62.8834, 58.5762) (63.0278, 57.1856) (62.9672, 55.8024) (62.7246, 54.4561) (62.3294, 53.176) (61.8122, 51.9999) (61.1992, 50.9832) (60.5078, 50.205) (59.7465, 49.7471) (58.9155, 49.6738) (58.0066, 50.0094) (57.0046, 50.7228) (55.8959, 51.7447) (54.677, 52.9811) (53.3626, 54.3285) (51.9934, 55.6869) (50.6472, 56.9761) (49.4377, 58.1442) (48.4887, 59.1627) (48.0287, 59.852) (47.8881, 60.3034) (47.8887, 60.5789) (47.9123, 60.7108) knots 0 0 0 0 0 0 0.028571 0.057143 0.085714 0.114286 0.142857 0.171429 0.2 0.228571 0.257143 0.285714 0.314286 0.342857 0.371429 0.4 0.428571 0.457143 0.485714 0.514286 0.542857 0.571429 0.6 0.628571 0.657143 0.685714 0.714286 0.742857 0.771429 0.8 0.828571 0.857143 0.885714 0.914286 0.942857 0.971429 1 1 1 1 1 1
  spline S40 degree 5 poles (69.9115, 65.0567) (70.1958, 65.1629) (70.7736, 65.345) (71.6588, 65.524) (72.839, 65.5661) (74.2282, 65.2936) (75.4548, 64.717) (76.454, 63.8744) (77.1746, 62.8186) (77.5822, 61.615) (77.6584, 60.3374) (77.4003, 59.0634) (76.82, 57.8702) (75.9449, 56.8301) (74.817, 56.0067) (73.4924, 55.4517) (72.04, 55.2026) (70.5408, 55.2791) (69.0882, 55.68) (67.7858, 56.3799) (66.7357, 57.3343) (66.027, 58.4832) (65.7245, 59.7551) (65.8564, 61.0703) (66.4038, 62.3446) (67.3129, 63.495) (68.2669, 64.2556) (69.0681, 64.7076) (69.6273, 64.9504) (69.9115, 65.0567) knots 0 0 0 0 0 0 0.04 0.08 0.12 0.16 0.2 0.24 0.28 0.32 0.36 0.4 0.44 0.48 0.52 0.56 0.6 0.64 0.68 0.72 0.76 0.8 0.84 0.88 0.92 0.96 1 1 1 1 1 1
  spline S41 degree 5 poles (24.4337, 58.6904) (24.4356, 58.9513) (24.481, 59.5035) (24.6739, 60.4105) (25.1702, 61.7209) (26.1221, 63.3696) (27.3098, 64.8696) (28.6186, 66.0726) (29.9244, 66.8567) (31.1033, 67.1396) (32.0415, 66.8967) (32.6445, 66.1582) (32.8474, 64.9983) (32.6254, 63.5286) (32.0051, 61.8907) (31.0532, 60.2419) (29.8654, 58.742) (28.5567, 57.539) (27.2509, 56.7548) (26.072, 56.472) (25.1338, 56.7149) (24.6514, 57.3057) (24.4696, 57.9384) (24.4318, 58.4296) (24.4337, 58.6904) knots 0 0 0 0 0 0 0.05 0.1 0.15 0.2 0.25 0.3 0.35 0.4 0.45 0.5 0.55 0.6 0.65 0.7 0.75 0.8 0.85 0.9 0.95 1 1 1 1 1 1
  spline S42 degree 5 poles (13.035, 61.9962) (13.4783, 62.2883) (14.4113, 62.8574) (15.9296, 63.6608) (18.0903, 64.6038) (20.7196, 65.483) (22.9777, 65.9735) (24.612, 65.9978) (25.4591, 65.503) (25.5015, 64.4774) (24.8864, 62.9602) (23.8452, 61.0333) (22.6285, 58.8182) (21.4424, 56.4696) (20.3672, 54.1745) (19.3627, 52.1342) (18.3305, 50.5382) (17.159, 49.5382) (15.7719, 49.2253) (14.186, 49.5961) (12.5261, 50.5521) (10.9753, 51.9422) (9.7406, 53.5964) (9.0143, 55.3593) (8.9336, 57.13) (9.5693, 58.8529) (10.6516, 60.1672) (11.7516, 61.1052) (12.5917, 61.7042) (13.035, 61.9962) knots 0 0 0 0 0 0 0.04 0.08 0.12 0.16 0.2 0.24 0.28 0.32 0.36 0.4 0.44 0.48 0.52 0.56 0.6 0.64 0.68 0.72 0.76 0.8 0.84 0.88 0.92 0.96 1 1 1 1 1 1
  spline S43 degree 5 poles (90.7123, 63.2246) (90.9617, 63.4874) (91.4845, 63.9968) (92.3288, 64.7062) (93.5229, 65.5096) (94.9932, 66.1848) (96.3157, 66.4459) (97.3927, 66.2303) (98.1721, 65.5149) (98.6617, 64.331) (98.9042, 62.7524) (98.9552, 60.8876) (98.862, 58.8703) (98.638, 56.8519) (98.2531, 54.9911) (97.6607, 53.4379) (96.8178, 52.319) (95.7073, 51.7221) (94.3609, 51.6793) (92.8792, 52.1528) (91.4029, 53.0586) (90.0884, 54.2857) (89.0823, 55.7175) (88.4954, 57.2517) (88.3787, 58.8192) (88.7331, 60.3709) (89.36, 61.5675) (89.9882, 62.4205) (90.4629, 62.9619) (90.7123, 63.2246) knots 0 0 0 0 0 0 0.04 0.08 0.12 0.16 0.2 0.24 0.28 0.32 0.36 0.4 0.44 0.48 0.52 0.56 0.6 0.64 0.68 0.72 0.76 0.8 0.84 0.88 0.92 0.96 1 1 1 1 1 1
  spline S44 degree 5 poles (76.8718, 72.8109) (76.8823, 73.0863) (76.9201, 73.6349) (77.0261, 74.4502) (77.2591, 75.5194) (77.6711, 76.8223) (78.168, 78.0819) (78.7213, 79.272) (79.3211, 80.341) (79.9872, 81.2012) (80.753, 81.7521) (81.649, 81.9052) (82.6851, 81.6089) (83.8359, 80.8699) (85.051, 79.7365) (86.2626, 78.2868) (87.3935, 76.6153) (88.3652, 74.8207) (89.1059, 72.9916) (89.5576, 71.1981) (89.6789, 69.4965) (89.4487, 67.9312) (88.8699, 66.5379) (87.9725, 65.3456) (86.8197, 64.3803) (85.5049, 63.6657) (84.1335, 63.2206) (82.8068, 63.0568) (81.6065, 63.1771) (80.5759, 63.5729) (79.7119, 64.2227) (78.9878, 65.0958) (78.3694, 66.1549) (77.8347, 67.3588) (77.3895, 68.6653) (77.0558, 70.0335) (76.9003, 71.1483) (76.8567, 71.9827) (76.8612, 72.5356) (76.8718, 72.8109) knots 0 0 0 0 0 0 0.028571 0.057143 0.085714 0.114286 0.142857 0.171429 0.2 0.228571 0.257143 0.285714 0.314286 0.342857 0.371429 0.4 0.428571 0.457143 0.485714 0.514286 0.542857 0.571429 0.6 0.628571 0.657143 0.685714 0.714286 0.742857 0.771429 0.8 0.828571 0.857143 0.885714 0.914286 0.942857 0.971429 1 1 1 1 1 1
  spline S45 degree 5 poles (6.5174, 74.1234) (6.8625, 74.3811) (7.587, 74.8543) (8.7702, 75.4277) (10.4857, 75.8892) (12.6469, 75.9236) (14.5772, 75.4159) (16.0381, 74.403) (16.841, 72.9571) (16.8973, 71.1868) (16.2117, 69.2255) (14.8616, 67.2177) (12.983, 65.305) (10.7539, 63.6134) (8.3804, 62.2385) (6.0809, 61.2346) (4.0604, 60.6261) (2.4862, 60.4164) (1.4615, 60.5973) (1.0031, 61.157) (1.004, 62.0915) (1.2953, 63.3907) (1.721, 65.0203) (2.2273, 66.8998) (2.8602, 68.9069) (3.7108, 70.8973) (4.6451, 72.3549) (5.517, 73.3081) (6.1724, 73.8657) (6.5174, 74.1234) knots 0 0 0 0 0 0 0.04 0.08 0.12 0.16 0.2 0.24 0.28 0.32 0.36 0.4 0.44 0.48 0.52 0.56 0.6 0.64 0.68 0.72 0.76 0.8 0.84 0.88 0.92 0.96 1 1 1 1 1 1
  spline S46 degree 5 poles (57.3572, 70.7364) (57.3371, 70.9725) (57.3289, 71.4505) (57.4131, 72.1803) (57.7145, 73.1584) (58.3779, 74.3368) (59.2885, 75.4192) (60.4038, 76.3566) (61.6876, 77.1051) (63.1136, 77.6274) (64.6551, 77.895) (66.2786, 77.8906) (67.9355, 77.6096) (69.5547, 77.0631) (71.0337, 76.28) (72.2558, 75.3032) (73.109, 74.1848) (73.5058, 72.9815) (73.4002, 71.7509) (72.8109, 70.546) (71.8074, 69.415) (70.4894, 68.4011) (68.9695, 67.5417) (67.3554, 66.8686) (65.7288, 66.4069) (64.1454, 66.1751) (62.6452, 66.1839) (61.2587, 66.4354) (60.015, 66.9223) (58.9499, 67.627) (58.1096, 68.521) (57.6535, 69.3578) (57.4496, 70.0342) (57.3773, 70.5004) (57.3572, 70.7364) knots 0 0 0 0 0 0 0.033333 0.066667 0.1 0.133333 0.166667 0.2 0.233333 0.266667 0.3 0.333333 0.366667 0.4 0.433333 0.466667 0.5 0.533333 0.566667 0.6 0.633333 0.666667 0.7 0.733333 0.766667 0.8 0.833333 0.866667 0.9 0.933333 0.966667 1 1 1 1 1 1
  spline S47 degree 5 poles (18.6525, 89.3821) (18.879, 89.6415) (19.3713, 90.1099) (20.2179, 90.654) (21.5091, 91.0402) (23.2178, 90.9415) (24.8416, 90.2799) (26.2307, 89.104) (27.3072, 87.4891) (28.078, 85.5313) (28.6003, 83.3407) (28.9588, 81.0338) (29.2388, 78.727) (29.5017, 76.5291) (29.7567, 74.5346) (29.9423, 72.8169) (29.9643, 71.4297) (29.7281, 70.4057) (29.1696, 69.7579) (28.297, 69.477) (27.1779, 69.5405) (25.9025, 69.9265) (24.5471, 70.6292) (23.1658, 71.6573) (21.8037, 73.0194) (20.5034, 74.713) (19.3134, 76.7129) (18.2986, 78.9571) (17.543, 81.3401) (17.1328, 83.73) (17.1415, 85.9816) (17.5196, 87.5571) (18.0124, 88.5537) (18.426, 89.1227) (18.6525, 89.3821) knots 0 0 0 0 0 0 0.033333 0.066667 0.1 0.133333 0.166667 0.2 0.233333 0.266667 0.3 0.333333 0.366667 0.4 0.433333 0.466667 0.5 0.533333 0.566667 0.6 0.633333 0.666667 0.7 0.733333 0.766667 0.8 0.833333 0.866667 0.9 0.933333 0.966667 1 1 1 1 1 1
  spline S48 degree 5 poles (37.7837, 80.0951) (38.0198, 80.079) (38.4905, 80.0052) (39.1877, 79.7696) (40.0852, 79.208) (41.1287, 78.1261) (42.0779, 76.7172) (42.9231, 75.0507) (43.6574, 73.2088) (44.2737, 71.2817) (44.7619, 69.3644) (45.1054, 67.5523) (45.2861, 65.9332) (45.2897, 64.5778) (45.112, 63.5315) (44.765, 62.8036) (44.2809, 62.3617) (43.7229, 62.1132) (43.1639, 61.9443) (42.6557, 61.7742) (42.1904, 61.6245) (41.715, 61.5884) (41.174, 61.7447) (40.5454, 62.0866) (39.8311, 62.5564) (39.0471, 63.0826) (38.2116, 63.6218) (37.3394, 64.1792) (36.4461, 64.7875) (35.5509, 65.494) (34.6795, 66.3455) (33.8678, 67.3719) (33.1623, 68.577) (32.6129, 69.9438) (32.2675, 71.4368) (32.1657, 73.0054) (32.333, 74.587) (32.7749, 76.1094) (33.4698, 77.4946) (34.3759, 78.6637) (35.4381, 79.5429) (36.364, 79.9646) (37.0742, 80.102) (37.5477, 80.1112) (37.7837, 80.0951) knots 0 0 0 0 0 0 0.025 0.05 0.075 0.1 0.125 0.15 0.175 0.2 0.225 0.25 0.275 0.3 0.325 0.35 0.375 0.4 0.425 0.45 0.475 0.5 0.525 0.55 0.575 0.6 0.625 0.65 0.675 0.7 0.725 0.75 0.775 0.8 0.825 0.85 0.875 0.9 0.925 0.95 0.975 1 1 1 1 1 1
  spline S49 degree 5 poles (47.6013, 81.0859) (47.7696, 81.1543) (48.1253, 81.2334) (48.7116, 81.1812) (49.5764, 80.7974) (50.723, 79.9174) (51.8539, 78.7796) (52.8862, 77.5133) (53.7435, 76.1924) (54.3613, 74.8338) (54.6907, 73.4295) (54.7036, 71.9705) (54.3965, 70.4707) (53.7972, 68.9986) (52.9634, 67.6801) (51.9697, 66.6625) (50.8976, 66.0877) (49.825, 66.0635) (48.8142, 66.6297) (47.9114, 67.7578) (47.1511, 69.3663) (46.5598, 71.3309) (46.1588, 73.4955) (45.9683, 75.6818) (46.0066, 77.7043) (46.2852, 79.39) (46.7011, 80.3555) (47.1156, 80.8229) (47.4331, 81.0175) (47.6013, 81.0859) knots 0 0 0 0 0 0 0.04 0.08 0.12 0.16 0.2 0.24 0.28 0.32 0.36 0.4 0.44 0.48 0.52 0.56 0.6 0.64 0.68 0.72 0.76 0.8 0.84 0.88 0.92 0.96 1 1 1 1 1 1
  spline S50 degree 5 poles (88.1069, 84.3923) (88.2327, 84.4684) (88.5272, 84.5642) (89.0938, 84.5383) (90.0684, 84.1797) (91.5329, 83.2812) (93.1035, 82.052) (94.639, 80.6181) (96.0168, 79.0901) (97.1561, 77.5382) (98.012, 76.0027) (98.5672, 74.5106) (98.8235, 73.0907) (98.7953, 71.7869) (98.5007, 70.6775) (97.9578, 69.8759) (97.1881, 69.4945) (96.219, 69.6175) (95.0867, 70.2679) (93.8362, 71.4167) (92.5223, 72.991) (91.2098, 74.8828) (89.9739, 76.956) (88.902, 79.0537) (88.0904, 81.0081) (87.6284, 82.6583) (87.594, 83.6249) (87.7728, 84.1074) (87.9812, 84.3162) (88.1069, 84.3923) knots 0 0 0 0 0 0 0.04 0.08 0.12 0.16 0.2 0.24 0.28 0.32 0.36 0.4 0.44 0.48 0.52 0.56 0.6 0.64 0.68 0.72 0.76 0.8 0.84 0.88 0.92 0.96 1 1 1 1 1 1
  spline S51 degree 5 poles (95.3735, 91.3141) (95.5816, 91.4342) (96.0195, 91.5899) (96.7247, 91.561) (97.6848, 91.0012) (98.704, 89.5881) (99.3461, 87.7155) (99.4709, 85.6921) (99.0366, 83.8383) (98.1411, 82.4459) (96.969, 81.7486) (95.744, 81.8879) (94.6852, 82.883) (93.9547, 84.5747) (93.6456, 86.6563) (93.7933, 88.7535) (94.2595, 90.1389) (94.7706, 90.8696) (95.1653, 91.1941) (95.3735, 91.3141) knots 0 0 0 0 0 0 0.066667 0.133333 0.2 0.266667 0.333333 0.4 0.466667 0.533333 0.6 0.666667 0.733333 0.8 0.866667 0.933333 1 1 1 1 1 1
  spline S52 degree 5 poles (51.0301, 84.9596) (51.0552, 85.0783) (51.1247, 85.3003) (51.2854, 85.5865) (51.6032, 85.8778) (52.1401, 86.1118) (52.7824, 86.2412) (53.5027, 86.2859) (54.2827, 86.2562) (55.1068, 86.1542) (55.958, 85.9739) (56.8134, 85.7026) (57.6379, 85.3204) (58.3882, 84.8058) (59.0183, 84.1438) (59.486, 83.3329) (59.7574, 82.3919) (59.8144, 81.3702) (59.6556, 80.3438) (59.2923, 79.4004) (58.7465, 78.6277) (58.0478, 78.1002) (57.2311, 77.8657) (56.3342, 77.9353) (55.3967, 78.2917) (54.4593, 78.8954) (53.5625, 79.6916) (52.7457, 80.6162) (52.0462, 81.6028) (51.4976, 82.5871) (51.1269, 83.5109) (50.9874, 84.1631) (50.9741, 84.5881) (51.005, 84.8409) (51.0301, 84.9596) knots 0 0 0 0 0 0 0.033333 0.066667 0.1 0.133333 0.166667 0.2 0.233333 0.266667 0.3 0.333333 0.366667 0.4 0.433333 0.466667 0.5 0.533333 0.566667 0.6 0.633333 0.666667 0.7 0.733333 0.766667 0.8 0.833333 0.866667 0.9 0.933333 0.966667 1 1 1 1 1 1
  spline S53 degree 5 poles (63.0589, 87.3081) (63.2069, 87.4746) (63.5261, 87.7926) (64.0699, 88.2212) (64.9092, 88.688) (66.1086, 89.0999) (67.4173, 89.3538) (68.7937, 89.463) (70.1948, 89.4301) (71.5757, 89.2353) (72.8906, 88.8502) (74.0921, 88.249) (75.1316, 87.4222) (75.9598, 86.3873) (76.5261, 85.2052) (76.7835, 83.9697) (76.6958, 82.7852) (76.2443, 81.7496) (75.4346, 80.9341) (74.3038, 80.3651) (72.9125, 80.0373) (71.3382, 79.9249) (69.6682, 79.9938) (67.9932, 80.2122) (66.4001, 80.5649) (64.9671, 81.0528) (63.7619, 81.682) (62.838, 82.4548) (62.2317, 83.3614) (61.9594, 84.3694) (62.0141, 85.4178) (62.301, 86.2305) (62.6377, 86.7937) (62.9108, 87.1416) (63.0589, 87.3081) knots 0 0 0 0 0 0 0.033333 0.066667 0.1 0.133333 0.166667 0.2 0.233333 0.266667 0.3 0.333333 0.366667 0.4 0.433333 0.466667 0.5 0.533333 0.566667 0.6 0.633333 0.666667 0.7 0.733333 0.766667 0.8 0.833333 0.866667 0.9 0.933333 0.966667 1 1 1 1 1 1
  spline S54 degree 5 poles (19.4544, 97.9422) (19.5397, 97.7864) (19.6265, 97.447) (19.5088, 96.8524) (18.9052, 95.8651) (17.635, 94.2238) (16.1101, 92.1206) (14.5539, 89.5805) (13.0705, 86.7696) (11.6707, 83.9539) (10.3118, 81.4443) (8.9314, 79.5473) (7.4843, 78.5124) (5.9762, 78.4826) (4.505, 79.4349) (3.2297, 81.2173) (2.3294, 83.6005) (1.968, 86.3201) (2.2506, 89.1277) (3.2074, 91.8146) (4.8047, 94.2093) (6.9474, 96.1834) (9.4829, 97.6551) (12.2063, 98.5919) (14.8571, 99.0204) (17.1464, 99.013) (18.4794, 98.7255) (19.115, 98.3816) (19.3692, 98.0979) (19.4544, 97.9422) knots 0 0 0 0 0 0 0.04 0.08 0.12 0.16 0.2 0.24 0.28 0.32 0.36 0.4 0.44 0.48 0.52 0.56 0.6 0.64 0.68 0.72 0.76 0.8 0.84 0.88 0.92 0.96 1 1 1 1 1 1
  spline S55 degree 5 poles (45.6842, 92.9012) (45.8962, 92.6223) (46.2919, 92.0488) (46.8002, 91.1483) (47.3058, 89.9064) (47.6457, 88.4111) (47.6876, 87.0953) (47.4274, 86.0497) (46.8622, 85.295) (45.9949, 84.7822) (44.8426, 84.4411) (43.4445, 84.2205) (41.8669, 84.1196) (40.1872, 84.1666) (38.4807, 84.4053) (36.808, 84.8793) (35.1988, 85.6156) (33.647, 86.6141) (32.1309, 87.8526) (30.6286, 89.2886) (29.1353, 90.8622) (27.679, 92.4989) (26.341, 94.1111) (25.2583, 95.6034) (24.5844, 96.8858) (24.4564, 97.8863) (24.9631, 98.5618) (26.1041, 98.9142) (27.7952, 98.984) (29.9003, 98.8313) (32.2552, 98.5205) (34.694, 98.1041) (37.0759, 97.6049) (39.3044, 97.0071) (41.3154, 96.2754) (43.0712, 95.3691) (44.2569, 94.4811) (45.0199, 93.7221) (45.4722, 93.1801) (45.6842, 92.9012) knots 0 0 0 0 0 0 0.028571 0.057143 0.085714 0.114286 0.142857 0.171429 0.2 0.228571 0.257143 0.285714 0.314286 0.342857 0.371429 0.4 0.428571 0.457143 0.485714 0.514286 0.542857 0.571429 0.6 0.628571 0.657143 0.685714 0.714286 0.742857 0.771429 0.8 0.828571 0.857143 0.885714 0.914286 0.942857 0.971429 1 1 1 1 1 1